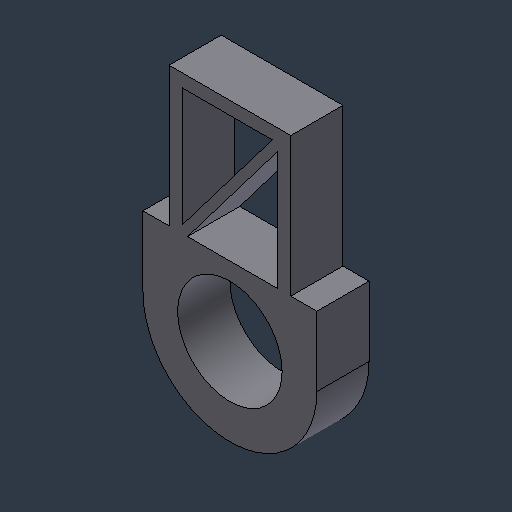
# Autodesk Inventor part: BLOCK,BEARING,ARM,ELEVATOR
Saved by Autodesk Inventor 2024.3 (Build 283343000, 343)
## iProperties
Category: _
Manager: _
ILogicPurgeVersion: 0.0.0.0
OnSaveVersion: 3.5.0.0
OnSaveAssembly: COREAutomationManager
Created: 2025-03-04
Part Number: BLOCK,BEARING,ARM,ELEVATOR
Checked By: 00
Engr Approved By: _
User Status: Work In Process
Material: Steel, MS
Description: STANDARD (mm)
Document SubType Name: Modeling
Mfg Approved By: John.Thibert
Designer: John.Thibert
Manufacturer: Standard
Standards Organization: Custom
Mass: 431.936 g
Surface Area: 190.473 cm^2
Volume: 54.9536 cm^3
Density: 7.86 g/cm^3
Appearance: Metal-Steel
CN_MASS: 0.43
CN_SERVICEABLE: _
FIRST_DESCRIPTION: _
SECOND_DESCRIPTION: _
THIRD_DESCRIPTION: _
ModelCat: Uncategorized
MaterialName: Steel, MS
Subject: _
Author: John.Thibert
Keywords: -
Revision Number: A
Autodesk Inventor part; units mm, degrees
ref_plane "YZ Plane" through (0, 0, 0) normal (1, 0, 0) x (0, 1, 0)
ref_plane "XZ Plane" through (0, 0, 0) normal (0, 1, 0) x (-1, 0, 0)
ref_plane "XY Plane" through (0, 0, 0) normal (0, 0, 1) x (1, 0, 0)
sketch "Sketch2" plane through (0, 0, 0) normal (0, 0, 1) x (1, 0, 0)
  line L0 (22.225, 0) -> (22.225, 50.8)
  line L1 (22.225, 50.8) -> (-22.225, 50.8)
  line L2 (-22.225, 50.8) -> (-22.225, 0)
  line L3 (22.225, 0) -> (31.75, 0)
  line L4 (31.75, 0) -> (31.75, -25.4)
  arc A0 (-31.75, -25.4) -> (31.75, -25.4) centre (0, -25.4) ccw
  line L5 (-31.75, -25.4) -> (-31.75, 0)
  line L6 (-31.75, 0) -> (-22.225, 0)
  line L7 (0, 72.39) -> (0, -78.74) construction
  line L8 (-44.45, 0) -> (44.45, 0) construction
  line L9 (-17.4625, 46.0375) -> (17.4625, 46.0375)
  line L10 (17.4625, 46.0375) -> (17.4625, 0)
  line L11 (17.4625, 0) -> (-17.4625, 0)
  line L12 (-17.4625, 0) -> (-17.4625, 46.0375)
  line L13 (-17.4625, 46.0375) -> (17.4625, 0) construction
  line L14 (17.4625, 46.0375) -> (-17.4625, 0) construction
  line L15 (17.4625, 43.4109) -> (-15.4699, 0)
  line L16 (15.4699, 46.0375) -> (-17.4625, 2.6266)
  point P0 (0, 0)
  point P1 (0, 50.8)
  point P2 (0, 23.0187)
  dimension "d0" = 44.45
  dimension "d1" = 50.8
  dimension "d2" = 25.4
  dimension "d3" = 31.75
  dimension "d6" = 4.7625
  dimension "d7" = 4.7625
  dimension "d8" = 1.5875
  constraints: 30 end point, 7 point on line, 5 perpendicular, 4 parallel, 3 midpoint, 2 collinear, 2 equal length, 2 horizontal, 2 point on circle, 2 tangent, 2 vertical, 1 centre point
  measures "d0" distance of L0.end L1.end
  measures "d1" distance of L1.end L2.end
  measures "d2" distance of L5.start L5.end
  measures "d3" radius of A0
  measures "d6" distance between parallel lines of L0 L10
  measures "d7" distance between parallel lines of L1 L9
  measures "d8" distance between parallel lines of L14 L16
extrude "Extrusion1" add sketch "Sketch2" along normal blind 19.05 contours L3 L4 A0 L5 L6 L2 L1 L0 | L9 L10 L15 L11 L12 L16
sketch "Sketch4" plane through (0, 0, 19.05) normal (0, 0, 1) x (1, 0, 0)
  arc A0 (-31.75, -25.4) -> (31.75, -25.4) centre (0, -25.4) ccw construction
  point P0 (0, 0)
  constraints: 1 coincident
hole "Hole1" at (0, -25.4, 19.05) direction (0, 0, -1) diameter 38.1 end through all
body "Solid1"
